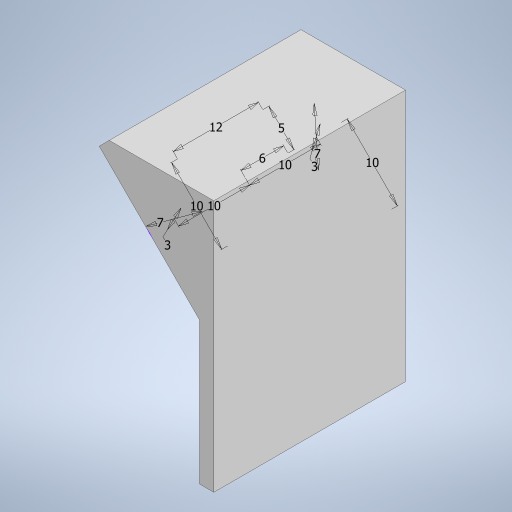
# Autodesk Inventor part: Time of Flight 4.0
Saved by Autodesk Inventor 2024 (Build 280153000, 153)
## iProperties
Created: 2024-04-01
Part Number: Time of Flight 4.0
Material: Generic
Document SubType Name: Modeling
Designer: olson
Density: 1 g/cm^3
Appearance: Default
Author: olson
Autodesk Inventor part; units mm, degrees
ref_plane "YZ Plane" through (0, 0, 0) normal (1, 0, 0) x (0, 1, 0)
ref_plane "XZ Plane" through (0, 0, 0) normal (0, 1, 0) x (-1, 0, 0)
ref_plane "XY Plane" through (0, 0, 0) normal (0, 0, 1) x (1, 0, 0)
sketch "Sketch1" plane through (0, 0, 0) normal (0, 0, 1) x (1, 0, 0)
  line L0 (0, 0) -> (14.1421, -14.1421)
  line L1 (0, 0) -> (20, 0) construction
  line L2 (14.1421, -14.1421) -> (15.5563, -12.7279)
  line L3 (15.5563, -12.7279) -> (1.4142, 1.4142)
  line L4 (1.4142, 1.4142) -> (0, 0)
  line L5 (1.4142, 1.4142) -> (15.5563, 1.4142)
  line L6 (14.1421, -14.1421) -> (14.1421, -34.1421)
  line L7 (14.1421, -34.1421) -> (16.1421, -34.1421)
  line L8 (16.1421, -34.1421) -> (16.1421, 1.4142)
  line L9 (16.1421, 1.4142) -> (15.5563, 1.4142)
  dimension "d0" = 20
  dimension "d1" = 45
  dimension "d2" = 2
  dimension "d3" = 20
  dimension "d4" = 20
  dimension "d6" = 2
  constraints: 20 end point, 4 perpendicular, 3 horizontal, 1 equal length, 1 vertical
  measures "d0" distance of L0.start L0.end
  measures "d1" angle of L0 L1
  measures "d2" distance of L0.end L2.end
  measures "d3" distance of L2.end L3.end
  measures "d4" distance of L0.end L6.end
  measures "d6" distance of L6.end L7.end
extrude "Extrusion1" add sketch "Sketch1" along normal blind 27
sketch "Sketch2" plane through (14.1421, -14.1421, 27) normal (-0.7071, -0.7071, 0) x (-0.7071, 0.7071, 0)
  line L0 (20, 27) -> (0, 27) projected
  line L1 (0, 27) -> (0, 0) projected
  line L2 (0, 27) -> (10, 27)
  line L3 (10, 27) -> (10, 13.5)
  line L4 (20, 27) -> (20, 0) projected
  line L5 (10, 13.5) -> (10, 19.5)
  line L6 (10, 19.5) -> (15, 19.5)
  line L7 (15, 19.5) -> (15, 7.5)
  line L8 (15, 7.5) -> (5, 7.5)
  line L9 (5, 7.5) -> (5, 19.5)
  line L10 (5, 19.5) -> (10, 19.5)
  line L11 (10, 13.5) -> (10, 23.5)
  circle A0 centre (10, 23.5) radius 1.5
  circle A1 centre (10, 23.5) radius 3.5
  line L12 (10, 13.5) -> (10, 3.5)
  circle A2 centre (10, 3.5) radius 1.5
  circle A3 centre (10, 3.5) radius 3.5
  dimension "d20" = 10
  dimension "d21" = 6
  dimension "d22" = 5
  dimension "d23" = 12
  dimension "d24" = 10
  dimension "d25" = 10
  dimension "d26" = 3
  dimension "d27" = 7
  dimension "d28" = 10
  dimension "d29" = 3
  dimension "d30" = 7
  constraints: 20 end point, 5 perpendicular, 4 centre point, 4 coincident, 3 point on line, 1 midpoint, 1 parallel, 1 vertical
  measures "d20" distance of L0.end L2.end
  measures "d21" distance of L3.end L5.end
  measures "d22" distance of L5.end L6.end
  measures "d23" distance of L6.end L7.end
  measures "d24" distance of L7.end L8.end
  measures "d25" distance of L3.end L11.end
  measures "d26" diameter of A0
  measures "d27" diameter of A1
  measures "d28" distance of L3.end L12.end
  measures "d29" diameter of A2
  measures "d30" diameter of A3
body "Solid1"
